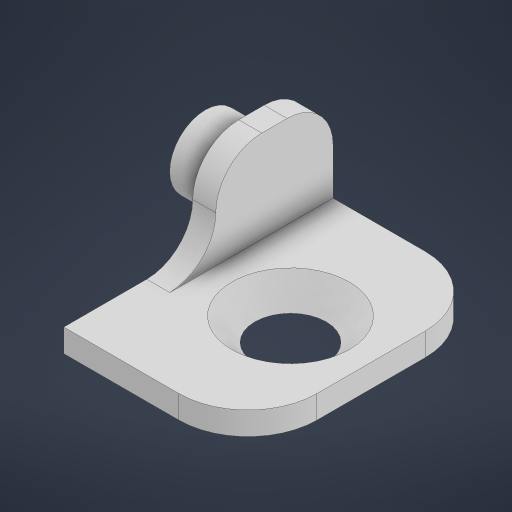
# Autodesk Inventor part: mocowanie_tofa
Saved by Autodesk Inventor 2024 (Build 280153000, 153)
## iProperties
Created: 2024-05-24
Part Number: mocowanie_tofa
Material: Generic
Document SubType Name: Modeling
Designer: Adam
Density: 1 g/cm^3
Appearance: Default
Mass: 0.10087 g
Surface Area: 2.61074 cm^2
Volume: 0.10087 cm^3
Author: Adam
Autodesk Inventor part; units mm, degrees
ref_plane "YZ Plane" through (0, 0, 0) normal (1, 0, 0) x (0, 1, 0)
ref_plane "XZ Plane" through (0, 0, 0) normal (0, 1, 0) x (-1, 0, 0)
ref_plane "XY Plane" through (0, 0, 0) normal (0, 0, 1) x (1, 0, 0)
sketch "Sketch1" plane through (0, 0, 0) normal (0, 0, 1) x (1, 0, 0)
  line L0 (0, 0) -> (8, 0)
  line L1 (8, 0) -> (8, 1)
  line L2 (8, 1) -> (1, 1)
  line L3 (1, 1) -> (1, 5)
  line L4 (1, 5) -> (0, 5)
  line L5 (0, 5) -> (0, 0)
  dimension "d0" = 8
  dimension "d1" = 5
  dimension "d2" = 1
  dimension "d8" = 1
  constraints: 12 end point, 5 perpendicular, 1 horizontal
  measures "d0" distance between parallel lines of L1 L5
  measures "d1" distance of L4.end L0.start
  measures "d2" distance between parallel lines of L2 L0
  measures "d8" distance between parallel lines of L3 L5
extrude "Extrusion1" add sketch "Sketch1" along normal blind 10.7
sketch "Sketch2" plane through (0, 0, 0) normal (-1, 0, 0) x (0, 0, 1)
  circle A0 centre (2.55, 2.55) radius 1.55
  line L0 (0, 0) -> (10.7, 0) projected
  line L1 (10.7, 5) -> (10.7, 0) projected
  line L2 (0, 5) -> (0, 0) projected
  dimension "d5" = 3.1
  dimension "d6" = 2.55
  dimension "d28" = 2.55
  constraints: 1 centre point
  measures "d5" diameter of A0
  measures "d6" distance from line of L0 A0.centre
  measures "d28" distance from line of L2 A0.centre
extrude "Extrusion2" add sketch "Sketch2" along normal blind 2
sketch "Sketch3" plane through (1, 1, 0) normal (0, 1, 0) x (1, 0, 0)
  line L0 (7, 0) -> (7, -10.7) projected
  line L1 (7, -10.7) -> (0, -10.7) projected
  point P0 (-1, 0)
  point P1 (3.5, -5.35)
  point P2 (3.5, -10.7)
  dimension "d11" = 3.5
  dimension "d12" = 5.35
  constraints: 1 midpoint
  measures "d11" distance from line of point (3.5, -5.35) L0
  measures "d12" distance of point (3.5, -10.7) point (3.5, -5.35)
hole "Hole1" at (4.5, 1, 5.35) direction (0, -1, 0) diameter 3.1 end through all
fillet "Fillet1" radius 3 2 edges at (8, 0.5, 0) (8, 0.5, 10.7)
fillet "Fillet3" radius 2 1 edges at (0.5, 5, 0)
sketch "Sketch5" plane through (0, 0, 10.7) normal (-1, 0, 0) x (0, 0, 1)
  line L0 (0, 1) -> (0, 5) projected
  line L1 (0, 5) -> (-5.6, 5)
  line L2 (-5.6, 5) -> (-5.6, 1)
  line L3 (-5.6, 1) -> (0, 1)
  line L4 (0, 1) -> (0, 5)
  circle A0 centre (-8.15, 2.55) radius 1.55 projected
  point P0 (-10.7, 0)
  dimension "d31" = 4
  dimension "d32" = 2.55
  constraints: 8 end point, 2 parallel, 1 horizontal, 1 perpendicular
  measures "d31" distance of L2.end L1.end
  measures "d32" distance from line of A0.centre L2
extrude "Extrusion4" cut sketch "Sketch5" against normal blind 1 contours L3 L2 L1 L0
fillet "Fillet4" radius 2 2 edges at (0.5, 1, 5.1) (0.5, 5, 5.1)
chamfer "Chamfer2" distance 1 angle 45 1 edges at (4.5, 1, 3.8) measured on face at (4.5, 1, 3.3)
body "Solid1"
